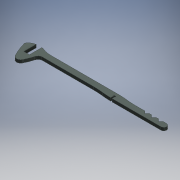
# Autodesk Inventor part: balancin
Saved by Autodesk Inventor 2016 (Build 200138000, 138)
## iProperties
Created: 2016-09-20
Part Number: balancin
Material: MDF Tablero de fibras de densidad media
Document SubType Name: Modeling
Designer: i95sa
Density: 0.8 g/cm^3
Appearance: Gris plomo - Pulido
Mass: 42.2014 g
Surface Area: 206.77 cm^2
Volume: 52.7517 cm^3
Author: i95sa
Autodesk Inventor part; units mm, degrees
ref_plane "YZ Plane" through (0, 0, 0) normal (1, 0, 0) x (0, 1, 0)
ref_plane "XZ Plane" through (0, 0, 0) normal (0, 1, 0) x (-1, 0, 0)
ref_plane "XY Plane" through (0, 0, 0) normal (0, 0, 1) x (1, 0, 0)
sketch "Boceto1" plane through (0, 0, 0) normal (0, 0, 1) x (1, 0, 0)
  line L0 (0, 1) -> (-2.2913, 1)
  line L1 (-2.2913, 1) -> (2.2913, 1)
  line L2 (0, 9) -> (-180.1018, 9)
  line L3 (-210, 0) -> (-210, 15)
  line L4 (-210, 15) -> (-210, -18)
  line L5 (-210, -18) -> (-225, -18)
  line L6 (-225, -18) -> (-225, 15)
  line L7 (-49.5857, -6) -> (-188.682, -6)
  line L8 (1.75, -9) -> (132.5, -9)
  arc A0 (-204.1562, 13.7709) -> (-210, 15) centre (-209.8984, 0.976) ccw
  arc A1 (-204.1562, 13.7709) -> (-180.1018, 9) centre (-180.1018, 72.0251) ccw
  arc A2 (-239.7755, 7.51) -> (-242.7743, 0.4952) centre (-233.8888, 0.8451) ccw
  arc A3 (-225, 15) -> (-239.7755, 7.51) centre (-217.9806, -17.166) ccw
  arc A4 (-242.7743, 0.4952) -> (-227.0984, -38.9645) centre (-54.9857, 52.2529) ccw
  arc A5 (-207.0119, -36.2943) -> (-198.7766, -14.633) centre (-315.3603, 17.2942) ccw
  arc A6 (-188.682, -6) -> (-198.7766, -14.633) centre (-186.7113, -18.5226) ccw
  arc A7 (-227.0984, -38.9645) -> (-208.1073, -38.6004) centre (-217.6949, -33.9808) ccw
  arc A8 (-25, -7.5) -> (-50, -6) centre (-49.7928, -211.6306) ccw
  arc A9 (-25, -7.5) -> (-1.75, -8.9981) centre (-0.6579, 189.118) ccw
  arc A10 (25, 7.51) -> (50, 6) centre (49.4872, 205.2229) ccw
  arc A11 (25, 7.51) -> (0, 9) centre (0.9036, -186.3114) ccw
  arc A12 (132.5, -9) -> (132.5, 6) centre (132.5, -1.5) ccw
  line L9 (132.5, 6) -> (122.5, 6)
  line L10 (122.5, 6) -> (116.5, 0)
  line L11 (110.5, 6) -> (116.5, 0)
  line L12 (110.5, 6) -> (104.5, 6)
  line L13 (92.5, 6) -> (86.5, 6)
  line L14 (74.966, 6) -> (74.5, 6)
  line L15 (104.5, 6) -> (98.5, 0)
  line L16 (98.5, 0) -> (92.5, 6)
  line L17 (86.5, 6) -> (80.5, 0)
  line L18 (74.5, 6) -> (80.5, 0)
  line L19 (132.5, 6) -> (122.5, 6)
  line L20 (110.5, 6) -> (104.5, 6)
  line L21 (92.5, 6) -> (86.5, 6)
  line L22 (74.5, 6) -> (50, 6)
  line L23 (-225, -18) -> (-210, -18)
  line L24 (-208.1073, -38.6004) -> (-207.0119, -36.2943)
  line L25 (1.75, -1.7854) -> (1.75, -9)
  line L26 (-1.75, -1.7854) -> (-1.75, -8.9981)
  arc A13 (-2.2913, 1) -> (-1.75, -1.7854) centre (0, 0) ccw
  arc A14 (1.75, -1.7854) -> (2.2913, 1) centre (0, 0) ccw
  constraints: 54 end point, 32 point on circle, 15 centre point, 6 perpendicular, 3 tangent, 2 horizontal, 2 vertical, 1 coincident, 1 parallel, 1 point on line
extrude "Extrusión2" add sketch "Boceto1" along normal blind 8
